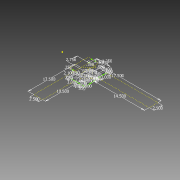
# Autodesk Inventor part: Laser_Holder
Saved by Autodesk Inventor 2013 (Build 170138000, 138)
## iProperties
Created: 2015-03-30
Part Number: Laser_Holder
Material: Generic
Document SubType Name: Modeling
Designer: Pat
Density: 1 g/cm^3
Author: Pat
Autodesk Inventor part; units mm, degrees
ref_plane "YZ Plane" through (0, 0, 0) normal (1, 0, 0) x (0, 1, 0)
ref_plane "XZ Plane" through (0, 0, 0) normal (0, 1, 0) x (-1, 0, 0)
ref_plane "XY Plane" through (0, 0, 0) normal (0, 0, 1) x (1, 0, 0)
sketch "Sketch1" plane through (0, 0, 0) normal (0, 1, 0) x (-1, 0, 0)
  line L0 (-203.3861, 74.2822) -> (-125.9161, 74.2822) construction
  line L1 (-125.9161, 74.2822) -> (-125.9161, -61.6078) construction
  line L2 (-125.9161, -61.6078) -> (-203.3861, -61.6078) construction
  line L3 (-203.3861, -61.6078) -> (-203.3861, 74.2822) construction
  line L4 (-203.3861, 74.2822) -> (-266.8861, 74.2822) construction
  line L5 (-164.6511, 373.4543) -> (-228.1511, 373.4543) construction
  line L6 (-228.1511, 373.4543) -> (-228.1511, 106.7543) construction
  line L7 (-228.1511, 106.7543) -> (-299.9932, 34.9122) construction
  line L8 (-299.9932, 34.9122) -> (-668.2932, 34.9122) construction
  line L9 (-668.2932, 34.9122) -> (-668.2932, -28.5878) construction
  line L10 (-668.2932, -28.5878) -> (-223.7932, -28.5878) construction
  line L11 (-223.7932, -28.5878) -> (-164.6511, 30.5543) construction
  line L12 (-164.6511, 30.5543) -> (-164.6511, 373.4543) construction
  line L13 (-264.0722, 70.8332) -> (-194.2222, 0.9832) construction
  line L14 (-266.8861, 74.2822) -> (-266.8861, 48.8822) construction
  line L15 (-266.8861, 48.8822) -> (-203.3861, -14.6178) construction
  line L16 (-266.8861, 68.0193) -> (-260.6232, 74.2822) construction
  circle A0 centre (-251.4998, 58.2609) radius 2.54
  circle A1 centre (-215.5788, 22.3399) radius 1.7653
  line L17 (-264.6511, 135.2422) -> (-188.4511, 135.2422)
  line L18 (-188.4511, 135.2422) -> (-188.4511, 81.9022)
  line L19 (-188.4511, 81.9022) -> (-264.6511, 81.9022)
  line L20 (-264.6511, 81.9022) -> (-264.6511, 135.2422)
  circle A2 centre (-164.6511, -28.5878) radius 4.9213 construction
  line L21 (-164.6511, 30.5543) -> (-164.6511, -28.5878) construction
  line L22 (-164.6511, -28.5878) -> (-223.7932, -28.5878) construction
  line L23 (-264.6511, 136.5122) -> (-187.1811, 136.5122)
  line L24 (-187.1811, 136.5122) -> (-187.1811, 80.6322)
  line L25 (-187.1811, 80.6322) -> (-264.6511, 80.6322)
  line L26 (-264.6511, 80.6322) -> (-264.6511, 136.5122)
  line L27 (-289.7461, 41.4122) -> (-236.4061, 41.4122)
  line L28 (-236.4061, 41.4122) -> (-236.4061, -34.7878)
  line L29 (-236.4061, -34.7878) -> (-289.7461, -34.7878)
  line L30 (-289.7461, -34.7878) -> (-289.7461, 41.4122)
  line L31 (-291.0161, 42.6822) -> (-235.1361, 42.6822)
  line L32 (-235.1361, 42.6822) -> (-235.1361, -36.0578)
  line L33 (-235.1361, -36.0578) -> (-291.0161, -36.0578)
  line L34 (-291.0161, -36.0578) -> (-291.0161, 42.6822)
  line L35 (-235.1361, -5.4793) -> (-209.7361, 19.9207)
  line L36 (-209.7361, 19.9207) -> (-209.7361, 80.6322)
  line L37 (-264.6511, 136.5122) -> (-264.6511, 80.6322)
  line L38 (-264.6511, 81.9022) -> (-264.6511, 135.2422)
  line L39 (-264.6511, 80.6322) -> (-264.6511, 136.5122)
  line L40 (-265.9211, 135.2422) -> (-297.6711, 135.2422)
  line L41 (-297.6711, 135.2422) -> (-297.6711, 81.9022)
  line L42 (-297.6711, 81.9022) -> (-265.9211, 81.9022)
  line L43 (-265.9211, 81.9022) -> (-265.9211, 135.2422)
  line L44 (-264.6511, 136.5122) -> (-298.9411, 136.5122)
  line L45 (-298.9411, 136.5122) -> (-298.9411, 80.6322)
  line L46 (-298.9411, 80.6322) -> (-264.6511, 80.6322)
  line L47 (-291.0161, 42.6822) -> (-298.9411, 80.6322)
  circle A3 centre (-278.6211, 114.9222) radius 3.175 construction
  point P0 (0, 0)
  point P1 (-177.3511, 74.2822)
  point P2 (-151.9511, 74.2822)
  point P3 (-177.3511, -61.6078)
  point P4 (-151.9511, -61.6078)
  dimension "d0" = 63.5
  dimension "d1" = 63.5
  dimension "d2" = 63.5
  dimension "d3" = 101.6
  dimension "d4" = 266.7
  dimension "d5" = 368.3
  dimension "d6" = 444.5
  dimension "d7" = 342.9
  dimension "d8" = 17.78
  dimension "d9" = 68.58
  dimension "d10" = 25.4
  dimension "d11" = 5.08
  dimension "d12" = 3.5306
  dimension "d14" = 76.2
  dimension "d15" = 9.8425
  dimension "d16" = 59.142
  dimension "d17" = 100
  dimension "d20" = 1.27
  dimension "d22" = 6.35
  dimension "d26" = 53.34
  dimension "d27" = 1.27
  dimension "d28" = 1.27
  dimension "d29" = 1.27
  dimension "d30" = 1.27
  dimension "d31" = 76.2
  dimension "d32" = 31.75
  dimension "d33" = 70
  dimension "d42" = 6.35
  dimension "d43" = 5.8426
  dimension "d44" = 5.842
  dimension "d50" = 31.75
  dimension "d51" = 1.27
  dimension "d52" = 1.27
  dimension "d53" = 53.34
  dimension "d54" = 1.27
  dimension "d55" = 1.27
  dimension "d71" = 6.35
  dimension "d72" = 20.32
  dimension "d73" = 12.7
  constraints: 97 end point, 19 parallel, 16 point on line, 15 perpendicular, 6 horizontal, 4 centre point, 4 collinear, 2 midpoint, 1 coincident
  measures "d0" distance of L4.start L4.end
  measures "d1" distance of L5.start L6.start
  measures "d2" distance of L9.start L10.start
  measures "d3" distance of L6.end L8.start
  measures "d4" distance of L6.start L6.end
  measures "d5" distance of L8.start L9.start
  measures "d6" distance of L11.start L10.start
  measures "d7" distance of L12.start L5.start
  measures "d8" distance from line of L7 point (-251.5, 58.261)
  measures "d9" distance from line of L7 point (-215.579, 22.34)
  measures "d10" distance of L4.end L15.start
  measures "d11" diameter of A0
  measures "d12" diameter of A1
  measures "d14" distance of L17.start L17.end
  measures "d15" diameter of A2
  measures "d16" distance of L11.start A2.centre
  measures "d17" distance from line of L22.start L20
  measures "d20" distance between parallel lines of L24 L18
  measures "d22" distance between parallel lines of L25 L0
  measures "d26" distance of L28.end L29.end
  measures "d27" distance between parallel lines of L32 L28
  measures "d28" distance between parallel lines of L30 L34
  measures "d29" distance between parallel lines of L33 L29
  measures "d30" distance between parallel lines of L31 L27
  measures "d31" distance between parallel lines of L29 L27
  measures "d32" distance between parallel lines of L3 L32
  measures "d33" distance from line of L27 A2.centre
  measures "d42" distance between parallel lines of L3 L36
  measures "d43" distance from line of L36 A1.centre
  measures "d44" distance from line of L35 point (-215.579, 22.34)
  measures "d50" distance of L40.start L40.end
  measures "d51" distance between parallel lines of L19 L25
  measures "d52" distance between parallel lines of L23 L17
  measures "d53" distance between parallel lines of L19 L17
  measures "d54" distance between parallel lines of L39 L43
  measures "d55" distance between parallel lines of L45 L41
  measures "d71" diameter of A3
  measures "d72" distance from line of A3.centre L40
  measures "d73" distance from line of A3.centre L43
extrude "Extrusion6" add sketch "Sketch1" along normal blind 5.08 contours L26 L23 L24 L25 L19 L18 L17 | L17 L18 L19 L20 | L20 L26 L46 L45 L44 | L25 L36 L35 L32 L31 L47 L46 | L31 L32 L33 L34 | L27 L28 L29 L30 | L43 L42 L41 L40
extrude "Extrusion7" add sketch "Sketch1" along normal blind 12.7 contours L26 L23 L24 L25 L19 L18 L17
extrude "Extrusion8" add sketch "Sketch1" along normal blind 12.7 contours L31 L32 L33 L34
extrude "Extrusion9" add sketch "Sketch1" along normal blind 15.24 contours L20 L26 L46 L45 L44
sketch "Sketch6" plane through (0, 12.7, 0) normal (0, 1, 0) x (1, 0, 0)
  line L0 (187.1811, -80.6322) -> (187.1811, -136.5122) projected
  line L1 (188.4511, -81.9022) -> (187.1811, -81.9022)
  line L2 (187.1811, -81.9022) -> (187.1811, -135.2422)
  line L3 (187.1811, -135.2422) -> (188.4511, -135.2422)
  line L4 (188.4511, -135.2422) -> (188.4511, -81.9022)
  point P0 (0, 0)
  constraints: 8 end point, 2 parallel, 1 horizontal, 1 perpendicular, 1 point on line
extrude "Extrusion11" cut sketch "Sketch6" against normal blind 25.4
sketch "Sketch7" plane through (0, 12.7, 0) normal (0, 1, 0) x (1, 0, 0)
  line L0 (291.0161, 36.0578) -> (235.1361, 36.0578) projected
  line L1 (236.4061, 34.7878) -> (289.7461, 34.7878)
  line L2 (289.7461, 34.7878) -> (289.7461, 36.0578)
  line L3 (289.7461, 36.0578) -> (236.4061, 36.0578)
  line L4 (236.4061, 36.0578) -> (236.4061, 34.7878)
  point P0 (0, 0)
  constraints: 8 end point, 2 parallel, 1 horizontal, 1 perpendicular, 1 point on line
extrude "Extrusion12" cut sketch "Sketch7" against normal blind 25.4
sketch "Sketch8" plane through (0, 5.08, 0) normal (0, 1, 0) x (1, 0, 0)
  line L0 (265.9211, -81.9022) -> (265.9211, -135.2422) projected
  line L1 (265.9211, -135.2422) -> (297.6711, -135.2422) projected
  line L2 (297.6711, -135.2422) -> (297.6711, -81.9022) projected
  line L3 (297.6711, -81.9022) -> (265.9211, -81.9022) projected
  line L4 (278.6211, -91.4272) -> (284.9711, -91.4272)
  line L5 (288.1461, -94.6022) -> (288.1461, -122.5422)
  line L6 (284.9711, -125.7172) -> (278.6211, -125.7172)
  line L7 (275.4461, -122.5422) -> (275.4461, -94.6022)
  arc A0 (278.6211, -91.4272) -> (275.4461, -94.6022) centre (278.6211, -94.6022) ccw
  arc A1 (288.1461, -94.6022) -> (284.9711, -91.4272) centre (284.9711, -94.6022) ccw
  arc A2 (284.9711, -125.7172) -> (288.1461, -122.5422) centre (284.9711, -122.5422) ccw
  arc A3 (275.4461, -122.5422) -> (278.6211, -125.7172) centre (278.6211, -122.5422) ccw
  point P0 (0, 0)
  point P1 (275.4461, -91.4272)
  point P2 (288.1461, -125.7172)
  point P3 (288.1461, -91.4272)
  point P4 (275.4461, -125.7172)
  dimension "d74" = 9.525
  dimension "d75" = 9.525
  dimension "d76" = 9.525
  dimension "d77" = 9.525
  dimension "d115" = 3.175
  constraints: 8 end point, 8 point on circle, 8 point on line, 8 tangent, 4 centre point, 3 equal radius, 2 parallel, 1 horizontal, 1 perpendicular
  measures "d74" distance between parallel lines of L3 L4
  measures "d75" distance between parallel lines of L5 L2
  measures "d76" distance between parallel lines of L7 L0
  measures "d77" distance between parallel lines of L1 L6
  measures "d115" radius of A0
extrude "Extrusion13" cut sketch "Sketch8" against normal blind 25.4 contours L4 A1 L5 A2 L6 A3 L7 A0
sketch "Sketch9" plane through (0, 5.08, 0) normal (0, 1, 0) x (1, 0, 0)
  line L0 (264.6511, -135.2422) -> (264.6511, -81.9022) projected
  line L1 (188.4511, -81.9022) -> (188.4511, -135.2422) projected
  line L2 (255.1261, -94.6022) -> (255.1261, -122.5422)
  line L3 (197.9761, -122.5422) -> (197.9761, -94.6022)
  line L4 (223.3761, -94.6022) -> (223.3761, -122.5422)
  line L5 (229.7261, -94.6022) -> (229.7261, -122.5422)
  line L6 (201.1511, -91.4272) -> (220.2011, -91.4272)
  line L7 (232.9011, -91.4272) -> (251.9511, -91.4272)
  line L8 (251.9511, -125.7172) -> (232.9011, -125.7172)
  line L9 (220.2011, -125.7172) -> (201.1511, -125.7172)
  arc A0 (201.1511, -91.4272) -> (197.9761, -94.6022) centre (201.1511, -94.6022) ccw
  arc A1 (223.3761, -94.6022) -> (220.2011, -91.4272) centre (220.2011, -94.6022) ccw
  arc A2 (197.9761, -122.5422) -> (201.1511, -125.7172) centre (201.1511, -122.5422) ccw
  arc A3 (220.2011, -125.7172) -> (223.3761, -122.5422) centre (220.2011, -122.5422) ccw
  arc A4 (229.7261, -122.5422) -> (232.9011, -125.7172) centre (232.9011, -122.5422) ccw
  arc A5 (232.9011, -91.4272) -> (229.7261, -94.6022) centre (232.9011, -94.6022) ccw
  arc A6 (255.1261, -94.6022) -> (251.9511, -91.4272) centre (251.9511, -94.6022) ccw
  arc A7 (251.9511, -125.7172) -> (255.1261, -122.5422) centre (251.9511, -122.5422) ccw
  point P0 (0, 0)
  point P1 (197.9761, -91.4272)
  point P2 (255.1261, -125.7172)
  point P3 (255.1261, -91.4272)
  point P4 (197.9761, -125.7172)
  point P5 (223.3761, -91.4272)
  point P6 (223.3761, -125.7172)
  point P7 (229.7261, -91.4272)
  point P8 (229.7261, -125.7172)
  dimension "d80" = 9.525
  dimension "d82" = 9.525
  dimension "d84" = 25.4
  dimension "d85" = 25.4
  dimension "d116" = 3.175
  constraints: 16 end point, 16 point on circle, 16 point on line, 16 tangent, 8 centre point, 7 equal radius, 4 equal length, 1 perpendicular
  measures "d80" distance between parallel lines of L1 L3
  measures "d82" distance between parallel lines of L0 L2
  measures "d84" distance between parallel lines of L4 L3
  measures "d85" distance between parallel lines of L2 L5
  measures "d116" radius of A0
extrude "Extrusion14" cut sketch "Sketch9" against normal blind 25.4
sketch "Sketch10" plane through (0, 5.08, 0) normal (0, 1, 0) x (1, 0, 0)
  line L0 (236.4061, -41.4122) -> (289.7461, -41.4122) projected
  line L1 (289.7461, 34.7878) -> (236.4061, 34.7878) projected
  line L2 (249.1061, 25.2628) -> (277.0461, 25.2628)
  line L3 (277.0461, -31.8872) -> (249.1061, -31.8872)
  line L4 (249.1061, -0.1372) -> (277.0461, -0.1372)
  line L5 (249.1061, -6.4872) -> (277.0461, -6.4872)
  line L6 (188.4511, -135.2422) -> (264.6511, -135.2422) projected
  line L7 (280.2211, 22.0878) -> (280.2211, 3.0378)
  line L8 (280.2211, -9.6622) -> (280.2211, -28.7122)
  line L9 (245.9311, -28.7122) -> (245.9311, -9.6622)
  line L10 (245.9311, 3.0378) -> (245.9311, 22.0878)
  arc A0 (245.9311, 3.0378) -> (249.1061, -0.1372) centre (249.1061, 3.0378) ccw
  arc A1 (249.1061, 25.2628) -> (245.9311, 22.0878) centre (249.1061, 22.0878) ccw
  arc A2 (280.2211, 22.0878) -> (277.0461, 25.2628) centre (277.0461, 22.0878) ccw
  arc A3 (277.0461, -0.1372) -> (280.2211, 3.0378) centre (277.0461, 3.0378) ccw
  arc A4 (280.2211, -9.6622) -> (277.0461, -6.4872) centre (277.0461, -9.6622) ccw
  arc A5 (249.1061, -6.4872) -> (245.9311, -9.6622) centre (249.1061, -9.6622) ccw
  arc A6 (245.9311, -28.7122) -> (249.1061, -31.8872) centre (249.1061, -28.7122) ccw
  arc A7 (277.0461, -31.8872) -> (280.2211, -28.7122) centre (277.0461, -28.7122) ccw
  point P0 (0, 0)
  point P1 (245.9311, 25.2628)
  point P2 (280.2211, -31.8872)
  point P3 (280.2211, 25.2628)
  point P4 (245.9311, -31.8872)
  point P5 (245.9311, -0.1372)
  point P6 (280.2211, -0.1372)
  point P7 (245.9311, -6.4872)
  point P8 (280.2211, -6.4872)
  dimension "d88" = 9.525
  dimension "d91" = 9.525
  dimension "d92" = 25.4
  dimension "d93" = 25.4
  dimension "d117" = 3.175
  constraints: 16 end point, 16 point on circle, 16 point on line, 16 tangent, 8 centre point, 7 equal radius, 5 equal length, 1 horizontal, 1 perpendicular
  measures "d88" distance between parallel lines of L1 L2
  measures "d91" distance between parallel lines of L0 L3
  measures "d92" distance between parallel lines of L2 L4
  measures "d93" distance between parallel lines of L3 L5
  measures "d117" radius of A0
extrude "Extrusion15" cut sketch "Sketch10" against normal blind 25.4
sketch "Sketch11" plane through (0, 5.08, 0) normal (0, 1, 0) x (1, 0, 0)
  line L0 (209.7361, -80.6322) -> (298.9411, -80.6322) projected
  line L1 (298.9411, -80.6322) -> (291.0161, -42.6822) projected
  line L2 (291.0161, -42.6822) -> (235.1361, -42.6822) projected
  line L3 (235.1361, -42.6822) -> (235.1361, 5.4793) projected
  line L4 (235.1361, 5.4793) -> (209.7361, -19.9207) projected
  line L5 (209.7361, -19.9207) -> (209.7361, -80.6322) projected
  circle A0 centre (215.5788, -22.3399) radius 1.7653 projected
  circle A1 centre (251.4998, -58.2609) radius 2.54 projected
  line L6 (265.0899, -49.0322) -> (280.0312, -49.0322)
  line L7 (283.1392, -51.5582) -> (287.086, -70.4582)
  line L8 (283.9781, -74.2822) -> (266.5077, -74.2822)
  line L9 (261.982, -51.5579) -> (258.0336, -70.4579)
  line L10 (261.1415, -74.2822) -> (266.5077, -74.2822)
  line L11 (243.5469, -52.8565) -> (239.5985, -71.7565)
  line L12 (236.4906, -74.2822) -> (222.4361, -74.2822)
  line L13 (219.2611, -71.1072) -> (219.2611, -52.2072)
  line L14 (222.4361, -49.0322) -> (240.439, -49.0322)
  line L15 (229.4211, -42.6822) -> (222.4361, -42.6822)
  line L16 (219.2611, -39.5072) -> (219.2611, -26.5422)
  line L17 (232.5961, -13.5971) -> (232.5961, -39.5072)
  line L18 (235.1361, -42.6822) -> (291.0161, -42.6822) projected
  line L19 (221.1541, -21.9731) -> (230.4281, -12.6991)
  line L20 (232.5961, -10.531) -> (232.5961, -13.2072)
  line L21 (188.4511, -135.2422) -> (264.6511, -135.2422) projected
  arc A2 (243.5469, -52.8565) -> (240.439, -49.0322) centre (240.439, -52.2072) ccw
  arc A3 (222.4361, -49.0322) -> (219.2611, -52.2072) centre (222.4361, -52.2072) ccw
  arc A4 (219.2611, -71.1072) -> (222.4361, -74.2822) centre (222.4361, -71.1072) ccw
  arc A5 (236.4906, -74.2822) -> (239.5985, -71.7565) centre (236.4906, -71.1072) ccw
  arc A6 (258.0336, -70.4579) -> (261.1415, -74.2822) centre (261.1415, -71.1072) ccw
  arc A7 (265.0899, -49.0322) -> (261.982, -51.5579) centre (265.0899, -52.2072) ccw
  arc A8 (283.1392, -51.5582) -> (280.0312, -49.0322) centre (280.0312, -52.2072) ccw
  arc A9 (283.9781, -74.2822) -> (287.086, -70.4582) centre (283.9781, -71.1072) ccw
  arc A10 (229.4211, -42.6822) -> (232.5961, -39.5072) centre (229.4211, -39.5072) ccw
  arc A11 (219.2611, -39.5072) -> (222.4361, -42.6822) centre (222.4361, -39.5072) ccw
  arc A12 (232.5961, -13.5971) -> (230.4281, -12.6991) centre (231.3261, -13.5971) ccw
  line L22 (221.1541, -21.9731) -> (220.3771, -22.7501)
  line L23 (219.2611, -25.4442) -> (219.2611, -26.5422)
  arc A13 (220.3771, -22.7501) -> (219.2611, -25.4442) centre (223.0711, -25.4442) ccw
  point P0 (0, 0)
  point P1 (282.6117, -49.0322)
  point P2 (287.8846, -74.2822)
  point P3 (262.5097, -49.0322)
  point P4 (257.2347, -74.2822)
  point P5 (244.3458, -49.0322)
  point P6 (239.0708, -74.2822)
  point P7 (219.2611, -74.2822)
  point P8 (219.2611, -49.0322)
  point P9 (232.5961, -42.6822)
  point P10 (219.2611, -42.6822)
  dimension "d96" = 6.35
  dimension "d97" = 9.525
  dimension "d98" = 6.35
  dimension "d100" = 101.795
  dimension "d101" = 101.8
  dimension "d102" = 6.35
  dimension "d103" = 9.525
  dimension "d104" = 6.35
  dimension "d105" = 6.35
  dimension "d106" = 6.35
  dimension "d108" = 2.54
  dimension "d111" = 9.525
  dimension "d118" = 3.175
  dimension "d119" = 1.27
  dimension "d120" = 3.81
  dimension "d121" = 2.5347
  constraints: 32 end point, 24 point on circle, 24 tangent, 23 point on line, 12 centre point, 9 equal radius, 6 parallel, 5 collinear, 5 perpendicular
  measures "d96" distance between parallel lines of L2 L6
  measures "d97" distance between parallel lines of L1 L7
  measures "d98" distance between parallel lines of L8 L0
  measures "d100" angle of L7 L6
  measures "d101" angle of L9 L6
  measures "d102" distance edge to line of A1 L9
  measures "d103" distance between parallel lines of L13 L5
  measures "d104" distance between parallel lines of L0 L12
  measures "d105" distance between parallel lines of L2 L14
  measures "d106" distance edge to line of A1 L11
  measures "d108" distance between parallel lines of L17 L3
  measures "d111" distance between parallel lines of L4 L19
  measures "d118" radius of A2
  measures "d119" radius of A12
  measures "d120" radius of A13
extrude "Extrusion16" cut sketch "Sketch11" against normal blind 25.4 contours L6 A8 L7 A9 L8 L10 A6 L9 A7 | L11 A5 L12 A4 L13 A3 L14 A2 | L15 A11 L16 L23 A13 L22 L19 A12 L17 A10
body "Solid3"
